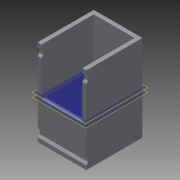
# Autodesk Inventor part: CarEngineHousing
Saved by Autodesk Inventor 2015 (Build 190159000, 159)
## iProperties
Created: 2016-03-26
Part Number: CarEngineHousing
Material: Generic
Document SubType Name: Modeling
Designer: Lee
Density: 1 g/cm^3
Appearance: Default
Author: Lee
Autodesk Inventor part; units mm, degrees
ref_plane "YZ Plane" through (0, 0, 0) normal (1, 0, 0) x (0, 1, 0)
ref_plane "XZ Plane" through (0, 0, 0) normal (0, 1, 0) x (-1, 0, 0)
ref_plane "XY Plane" through (0, 0, 0) normal (0, 0, 1) x (1, 0, 0)
sketch "Sketch1" plane through (0, 0, 0) normal (0, 0, 1) x (1, 0, 0)
  line L0 (0, 0) -> (1.6, 0)
  line L1 (1.6, 0) -> (1.6, 23.05)
  line L2 (1.6, 23.05) -> (0, 23.05)
  line L3 (0, 23.05) -> (0, 0)
  line L4 (0, 0) -> (19.97, 0)
  line L5 (19.97, 0) -> (19.97, 1.6)
  line L6 (19.97, 1.6) -> (0, 1.6)
  line L7 (0, 1.6) -> (0, 0)
  line L8 (0, 23.05) -> (19.97, 23.05)
  line L9 (19.97, 23.05) -> (19.97, 21.45)
  line L10 (19.97, 21.45) -> (0, 21.45)
  line L11 (0, 21.45) -> (0, 23.05)
  line L12 (19.97, 0) -> (18.37, 0)
  line L13 (18.37, 0) -> (18.37, 23.05)
  line L14 (18.37, 23.05) -> (19.97, 23.05)
  line L15 (19.97, 23.05) -> (19.97, 0)
  dimension "d0" = 1.6
  dimension "d1" = 1.6
  dimension "d2" = 1.6
  dimension "d3" = 1.6
  dimension "d4" = 19.85
  dimension "d5" = 16.77
  constraints: 32 end point, 8 parallel, 4 horizontal, 4 perpendicular, 2 point on line
  measures "d0" distance of L2.end L1.end
  measures "d1" distance of L5.end L4.end
  measures "d2" distance of L8.end L9.end
  measures "d3" distance of L13.end L14.end
  measures "d4" distance between parallel lines of L10 L6
  measures "d5" distance between parallel lines of L13 L1
extrude "Extrusion1" add sketch "Sketch1" along normal blind 35.48 contours L3 L6 L1 L0 | L1 L6 L13 L4 | L3 L10 L1 L6 | L13 L6 L5 L4 | L3 L2 L1 L10 | L1 L8 L13 L10 | L13 L10 L15 L6 | L13 L8 L9 L10
sketch "Sketch2" plane through (0, 0, 35.48) normal (0, 0, 1) x (1, 0, 0)
  line L0 (18.37, 21.45) -> (18.37, 1.6) projected
  line L1 (18.37, 1.6) -> (1.6, 1.6) projected
  line L2 (1.6, 1.6) -> (1.6, 21.45) projected
  line L3 (1.6, 21.45) -> (18.37, 21.45) projected
  line L4 (19.97, 23.05) -> (0, 23.05) projected
  line L5 (0, 23.05) -> (0, 0) projected
  line L6 (0, 0) -> (19.97, 0) projected
  line L7 (19.97, 0) -> (19.97, 23.05) projected
  line L8 (19.97, 0) -> (19.97, 23.05) projected
  line L9 (0, 0) -> (19.97, 0)
  line L10 (19.97, 0) -> (19.97, 1.6)
  line L11 (19.97, 1.6) -> (0, 1.6)
  line L12 (0, 1.6) -> (0, 0)
  line L13 (18.37, 1.6) -> (18.37, 0)
  line L14 (0, 0) -> (19.97, 0) projected
  line L15 (1.6, 1.6) -> (1.6, 0)
  line L16 (1.6, 1.6) -> (18.37, 1.6)
  line L17 (18.37, 1.6) -> (18.37, 0)
  line L18 (18.37, 0) -> (1.6, 0)
  line L19 (1.6, 0) -> (1.6, 1.6)
  constraints: 20 end point, 4 parallel, 3 point on line, 2 horizontal, 2 perpendicular
ref_plane "Work Plane1" through (0, 0, 16) normal (0, 0, -1) x (-1, 0, 0)
sketch "Sketch3" plane through (0, 0, 0) normal (-1, 0, 0) x (0, 0, 1)
  line L0 (0, 0) -> (35.48, 0) projected
  line L1 (1.7, 0) -> (2.5, 0.8)
  line L2 (1.7, 0) -> (2.8314, 0) construction
  line L3 (2.5, 0.8) -> (4.1, 0.8)
  line L4 (4.1, 0.8) -> (4.9, 0)
  line L5 (0, 23.05) -> (0, 0) projected
  point P0 (16, 0)
  dimension "d11" = 45
  dimension "d12" = 1.6
  dimension "d13" = 0.8
  dimension "d14" = 45
  dimension "d15" = 2.5
  constraints: 8 end point, 2 point on line, 1 equal length, 1 horizontal
  measures "d11" angle of L2 L1
  measures "d12" distance of L1.end L3.end
  measures "d13" distance between parallel lines of L0 L3
  measures "d14" angle of L0 L4
  measures "d15" distance from line of L5 L1.end
extrude "Extrusion3" cut sketch "Sketch3" against normal up to next
extrude "Extrusion4" cut sketch "Sketch2" against normal up to surface (19.48 mm away) contours L13 L6 L15 L1
ref_plane "Midway" through (0, 0, 17.74) normal (0, 0, -1) x (-1, 0, 0)
mirror "Mirror1" about plane through (0, 0, 17.74) normal (0, 0, -1) of "Extrusion3"
body "Solid1"
